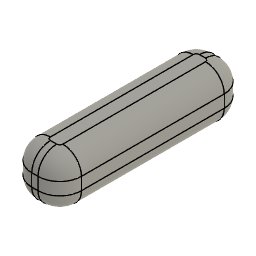
Microstir (Autodesk Fusion 360 archive; units mm, degrees)
design "Stirrer Bar"
Autodesk Fusion 360 part; units mm, degrees
sketch "Sketch1" plane through (0, 0, 0) normal (0, 1, 0) x (1, 0, 0)
  line L0 (0, 0) -> (8, 0)
  line L1 (8, 0) -> (8, -8)
  line L2 (8, -8) -> (0, -8)
  line L3 (0, -8) -> (0, 0)
  dimension "d1" = 8
  dimension "d2" = 8
  constraint horizontal L0
  constraint vertical L1
  constraint horizontal L2
  constraint vertical L3
  constraint coincident L0.start L3.end
  measures "d1" distance of L0.start L0.end
  measures "d2" distance of L0.start L2.end
extrude "Extrude1" add sketch "Sketch1" along normal blind 30
fillet "Fillet1" radius 3.5 4 edges at (8, 0, 4) (0, 0, 4) (0, 30, 4) (8, 30, 4)
fillet "Fillet2" radius 3 16 edges at (6.9749, 28.9749, 8) (4, 30, 8) (1.0251, 28.9749, 8) (0, 15, 8) (1.0251, 1.0251, 8) (4, 0, 8) (6.9749, 1.0251, 8) (8, 15, 8) (4, 30, 0) (1.0251, 28.9749, 0) (0, 15, 0) (1.0251, 1.0251, 0) (4, 0, 0) (6.9749, 1.0251, 0) (8, 15, 0) (6.9749, 28.9749, 0)

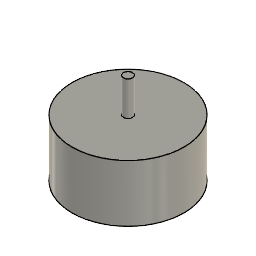
design "R300C DC Motor"
Autodesk Fusion 360 part; units mm, degrees
sketch "Sketch1" plane through (0, 0, 0) normal (0, 0, 1) x (1, 0, 0)
  circle A0 centre (0, 0) radius 12.25
  dimension "d1" = 24.5
  constraint coincident A0.centre origin
  measures "d1" diameter of A0
extrude "Extrude1" add sketch "Sketch1" along normal blind 12.5
sketch "Sketch2" plane through (0, 0, 12.5) normal (0, 0, 1) x (-1, 0, 0)
  circle A0 centre (0, 0) radius 12.25
  circle A1 centre (0, 0) radius 1
  dimension "d4" = 2
  constraint coincident A0.centre A1.centre
  measures "d4" diameter of A1
extrude "Extrude2" add sketch "Sketch2" along normal blind 7.5 contours A1

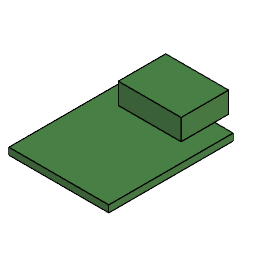
design "Charging Board"
Autodesk Fusion 360 part; units mm, degrees
sketch "Sketch1" plane through (0, 0, 0) normal (0, 0, 1) x (1, 0, 0)
  line L0 (-7.15, 8.9) -> (7.15, 8.9)
  line L1 (7.15, 8.9) -> (7.15, -8.9)
  line L2 (7.15, -8.9) -> (-7.15, -8.9)
  line L3 (-7.15, -8.9) -> (-7.15, 8.9)
  line L4 (-7.15, 8.9) -> (7.15, -8.9) construction
  line L5 (7.15, 8.9) -> (-7.15, -8.9) construction
  dimension "d13" = 14.3
  dimension "d14" = 17.8
  constraint horizontal L0
  constraint perpendicular L0 L1
  constraint parallel L0 L2
  constraint parallel L1 L3
  constraint coincident L4 origin
  constraint coincident L5 origin
  measures "d13" distance of L1.end L2.end
  measures "d14" distance of L0.end L1.end
extrude "Extrude5" add sketch "Sketch1" along normal blind 1
sketch "Sketch3" plane through (0, 0, 1) normal (0, 0, 1) x (-1, 0, 0)
  line L0 (7.15, 8.9) -> (-7.15, 8.9)
  line L1 (-7.15, 8.9) -> (-7.15, -8.9)
  line L2 (-7.15, -8.9) -> (7.15, -8.9)
  line L3 (7.15, -8.9) -> (7.15, 8.9)
  line L4 (0, -8.9) -> (0, -10.9)
  line L5 (4.5, -10.9) -> (-4.5, -10.9)
  line L6 (4.5, -10.9) -> (4.5, -4.1)
  line L7 (4.5, -4.1) -> (-4.5, -4.1)
  line L8 (-4.5, -4.1) -> (-4.5, -10.9)
  dimension "d17" = 2
  dimension "d18" = 4.5
  dimension "d19" = 9
  dimension "d20" = 6.8
  constraint midpoint L2 L4.start
  constraint perpendicular L2 L4
  constraint perpendicular L5 L6
  constraint perpendicular L6 L7
  constraint perpendicular L5 L8
  measures "d17" distance of L4.start L4.end
  measures "d18" distance of L4.end L5.start
  measures "d19" distance of L5.start L5.end
  measures "d20" distance of L5.start L6.end
extrude "Extrude6" add sketch "Sketch3" along normal blind 3 contours L2 L4 L5 L6 | L2 L6 L7 L8 | L2 L4 L5 L8

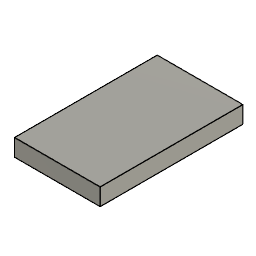
design "603048 Battery"
Autodesk Fusion 360 part; units mm, degrees
sketch "Sketch1" plane through (0, 0, 0) normal (0, 0, 1) x (1, 0, 0)
  line L0 (15, -25) -> (-15, -25)
  line L1 (-15, -25) -> (-15, 25)
  line L2 (-15, 25) -> (15, 25)
  line L3 (15, 25) -> (15, -25)
  line L4 (15, -25) -> (-15, 25) construction
  line L5 (-15, -25) -> (15, 25) construction
  line L6 (-15, 25) -> (-13.5, 25)
  line L7 (-13.5, 25) -> (-13.5, 26.5)
  line L8 (-13.5, 26.5) -> (-15, 26.5)
  line L9 (-15, 26.5) -> (-15, 25)
  line L10 (-13.5, 26.5) -> (-17, 26.5)
  line L11 (-17, 26.5) -> (-17, 25)
  line L12 (-17, 25) -> (-13.5, 25)
  line L13 (-13.5, 25) -> (-13.5, 26.5)
  line L14 (-13.5, 26.5) -> (-12, 26.5)
  line L15 (-12, 26.5) -> (-12, 25)
  line L16 (-12, 25) -> (-13.5, 25)
  line L17 (-13.5, 25) -> (-13.5, 26.5)
  dimension "d7" = 30
  dimension "d8" = 50
  constraint horizontal L0
  constraint perpendicular L0 L1
  constraint parallel L0 L2
  constraint parallel L1 L3
  constraint coincident L4 origin
  constraint coincident L5 origin
  constraint horizontal L6
  constraint vertical L7
  constraint horizontal L8
  constraint vertical L9
  constraint horizontal L10
  constraint vertical L11
  constraint horizontal L12
  constraint vertical L13
  constraint horizontal L14
  constraint vertical L15
  constraint horizontal L16
  constraint vertical L17
  constraint coincident L2 L15.end
  measures "d7" distance of L1.end L2.end
  measures "d8" distance of L0.end L1.end
extrude "Extrude3" add sketch "Sketch1" along normal blind 6 contours L0 L1 L2 L3 L6 L12 L16
extrude "Extrude4" add sketch "Sketch1" along normal blind 1.5 contours L2 L6 L7 L8 L9 L10 L12 L13 L17 | L9 L10 L11 L12 | L2 L7 L13 L14 L15 L16 L17
